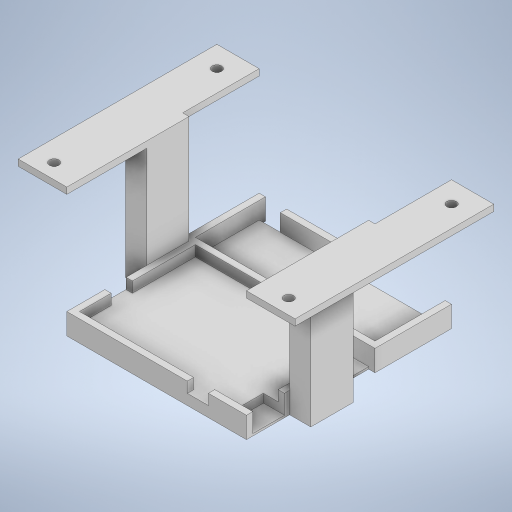
# Autodesk Inventor part: batter_pack_top
Saved by Autodesk Inventor 2023 (Build 270158000, 158)
## iProperties
Created: 2024-04-19
Part Number: batter_pack_top
Material: Genérico
Document SubType Name: Modeling
Designer: inigo
Density: 1 g/cm^3
Appearance: Valor por defecto
Author: inigo
Autodesk Inventor part; units mm, degrees
ref_plane "YZ Plane" through (0, 0, 0) normal (1, 0, 0) x (0, 1, 0)
ref_plane "XZ Plane" through (0, 0, 0) normal (0, 1, 0) x (-1, 0, 0)
ref_plane "XY Plane" through (0, 0, 0) normal (0, 0, 1) x (1, 0, 0)
sketch "Boceto1" plane through (0, 0, 0) normal (0, 1, 0) x (-1, 0, 0)
  line L0 (39.5, 42.5) -> (-39.5, 42.5)
  line L1 (-39.5, 42.5) -> (-39.5, -42.5)
  line L2 (-39.5, -42.5) -> (39.5, -42.5)
  line L3 (39.5, -42.5) -> (39.5, 42.5)
  line L4 (39.5, 42.5) -> (-39.5, -42.5) construction
  line L5 (-39.5, 42.5) -> (39.5, -42.5) construction
  line L6 (42.5, 45.5) -> (-42.5, 45.5)
  line L7 (-42.5, 45.5) -> (-42.5, -45.5)
  line L8 (-42.5, -45.5) -> (42.5, -45.5)
  line L9 (42.5, -45.5) -> (42.5, 45.5)
  point P0 (0, 0)
  point P1 (0, 0)
  dimension "d0" = 79
  dimension "d1" = 85
  dimension "d2" = 3
  constraints: 20 end point, 4 parallel, 2 midpoint, 2 perpendicular, 1 horizontal, 3 other
  measures "d0" distance of L2.end L1.end
  measures "d1" distance of L1.end L0.end
  measures "d2" distance between parallel lines of L3 L9
extrude "Extrusión1" add sketch "Boceto1" along normal blind 10 contours L3 L2 L1 L0 | L9 L8 L7 L6
sketch "Boceto2" plane through (0, 10, 0) normal (0, 1, 0) x (1, 0, 0)
  line L0 (-42.5, 45.5) -> (-42.5, -45.5)
  line L1 (42.5, -45.5) -> (-42.5, -45.5)
  line L2 (-42.5, -45.5) -> (-42.5, 45.5)
  line L3 (-42.5, 45.5) -> (42.5, 45.5)
  line L4 (42.5, 45.5) -> (42.5, -45.5)
  line L5 (42.5, -45.5) -> (-42.5, 45.5) construction
  line L6 (-42.5, -45.5) -> (42.5, 45.5) construction
  line L7 (-39.5, -42.5) -> (39.5, -42.5)
  line L8 (39.5, -42.5) -> (39.5, 42.5)
  line L9 (39.5, 42.5) -> (-39.5, 42.5)
  line L10 (-39.5, 42.5) -> (-39.5, -42.5)
  line L11 (0, -42.5) -> (0, -45.5)
  line L12 (-42.5, -45.5) -> (42.5, -45.5)
  line L13 (-15, -45.5) -> (15, -45.5)
  line L14 (15, -45.5) -> (15, -42.5)
  line L15 (15, -42.5) -> (-15, -42.5)
  line L16 (-15, -42.5) -> (-15, -45.5)
  line L17 (-15, -45.5) -> (15, -42.5) construction
  line L18 (15, -45.5) -> (-15, -42.5) construction
  line L19 (-65.3363, 15.3) -> (96.4695, 15.3)
  point P0 (0, 0)
  point P1 (0, -44)
  point P2 (39.5, 15.3)
  point P3 (-39.5, 15.3)
  dimension "d8" = 3
  dimension "d9" = 85
  dimension "d10" = 79
  dimension "d11" = 30
  dimension "d12" = 57.8
  constraints: 40 end point, 7 midpoint, 6 parallel, 3 horizontal, 3 perpendicular, 1 point on line, 3 other
  measures "d8" distance between parallel lines of L1 L7
  measures "d9" distance between parallel lines of L7 L9
  measures "d10" distance between parallel lines of L8 L10
  measures "d11" distance of L16.start L17.end
  measures "d12" distance between parallel lines of L7 L19
extrude "Extrusión2" cut sketch "Boceto2" against normal blind 5 contours L19 L8 L7 L10
sketch "Boceto3" plane through (0, 0, 0) normal (0, 1, 0) x (-1, 0, 0)
  line L0 (-42.5, 45.5) -> (-42.5, -15.3)
  line L1 (42.5, -45.5) -> (-42.5, -45.5)
  line L2 (-42.5, -45.5) -> (-42.5, -15.3)
  line L3 (-42.5, -15.3) -> (42.5, -15.3)
  line L4 (42.5, -15.3) -> (42.5, -45.5)
  line L5 (-45.5, -48.5) -> (45.5, -48.5)
  line L6 (45.5, -48.5) -> (45.5, -12.3)
  line L7 (45.5, -12.3) -> (-45.5, -12.3)
  line L8 (-45.5, -12.3) -> (-45.5, -48.5)
  line L9 (45.5, -15.3) -> (-45.5, -15.3)
  line L10 (-12.5, -48.5) -> (-12.5, -45.5)
  line L11 (-42.5, -45.5) -> (42.5, -45.5)
  line L12 (42.5, -45.5) -> (42.5, -48.5)
  line L13 (42.5, -15.3) -> (42.5, -12.3)
  line L14 (42.5, -45.5) -> (42.5, 45.5)
  line L15 (-42.5, -15.3) -> (-42.5, -12.3)
  line L16 (-42.5, 45.5) -> (-42.5, -45.5) projected
  line L17 (-42.5, -45.5) -> (-42.5, -48.5)
  line L18 (-42.5, -45.5) -> (42.5, -45.5) projected
  line L19 (2.5, -48.5) -> (32.5, -48.5)
  line L20 (32.5, -48.5) -> (32.5, -45.5)
  line L21 (32.5, -45.5) -> (2.5, -45.5)
  line L22 (2.5, -45.5) -> (2.5, -48.5)
  point P0 (0, 0)
  point P1 (0, 0)
  point P2 (-12.5, -47)
  point P3 (2.5, -45.5)
  point P4 (42.5, -47)
  point P5 (32.5, -47)
  dimension "d15" = 3
  dimension "d16" = 30
  dimension "d21" = 30
  dimension "d24" = 10
  constraints: 42 end point, 13 point on line, 6 parallel, 6 perpendicular, 3 midpoint, 2 horizontal, 3 other
  measures "d15" distance between parallel lines of L1 L5
  measures "d16" distance from line of L2 point (-12.5, -47)
  measures "d21" distance of L21.end L20.end
  measures "d24" distance of point (42.5, -47) point (32.5, -47)
extrude "Extrusión3" add sketch "Boceto3" along normal blind 10 contours L7 L13 L3 L0 | L0 L9 L8 L7 | L3 L4 L1 L2 | L2 L17 L5 L8 L9 | L7 L6 L9 L13 | L9 L6 L5 L12 L4 | L1 L20 L5 L22
sketch "Boceto4" plane through (0, 10, 0) normal (0, 1, 0) x (1, 0, 0)
  line L0 (-39.5, 15.3) -> (39.5, 15.3)
  line L1 (0, 15.3) -> (0, 45.5)
  line L2 (42.5, 45.5) -> (-42.5, 45.5)
  line L3 (-42.5, 45.5) -> (42.5, 45.5)
  line L4 (42.5, 45.5) -> (42.5, 15.3)
  line L5 (42.5, 15.3) -> (-42.5, 15.3)
  line L6 (-42.5, 15.3) -> (-42.5, 45.5)
  line L7 (-42.5, 45.5) -> (42.5, 15.3) construction
  line L8 (42.5, 45.5) -> (-42.5, 15.3) construction
  point P0 (0, 0)
  point P1 (0, 0)
  point P2 (0, 30.4)
  constraints: 18 end point, 5 midpoint, 2 parallel, 1 horizontal, 1 perpendicular
extrude "Extrusión4" cut sketch "Boceto4" against normal blind 8
sketch "Boceto5" plane through (-42.5, 0, 45.5) normal (-1, 0, 0) x (0, 0, 1)
  line L0 (-18, 10) -> (-28, 10)
  line L1 (-28, 10) -> (-28, 5)
  line L2 (-28, 5) -> (-18, 5)
  line L3 (-18, 5) -> (-18, 10)
  line L4 (-3, 5) -> (-57.8, 5) projected
  line L5 (-3, 10) -> (-3, 5) projected
  line L6 (-57.8, 10) -> (0, 10) projected
  point P0 (-45.5, 0)
  point P1 (-23, 5)
  dimension "d25" = 10
  dimension "d27" = 15
  dimension "d28" = 0
  dimension "d29" = 0
  constraints: 8 end point, 2 parallel, 1 horizontal, 1 perpendicular, 1 point on line
  measures "d25" distance of L2.end L1.end
  measures "d27" distance between parallel lines of L5 L3
  measures "d28" distance between parallel lines of L6 L0
  measures "d29" distance between parallel lines of L4 L2
extrude "Extrusión5" cut sketch "Boceto5" against normal blind 10 contours L3 L2 L1 L0
sketch "Boceto6" plane through (-42.5, 0, 45.5) normal (0, 0, 1) x (1, 0, 0)
  line L0 (67, 5) -> (57, 5)
  line L1 (57, 5) -> (57, 10)
  line L2 (57, 10) -> (67, 10)
  line L3 (67, 10) -> (67, 5)
  line L4 (82, 5) -> (3, 5) projected
  line L5 (85, 0) -> (85, 10) projected
  line L6 (0, 10) -> (85, 10) projected
  point P0 (42.5, 0)
  point P1 (62, 5)
  dimension "d32" = 10
  dimension "d33" = 18
  dimension "d34" = 0
  dimension "d35" = 0
  constraints: 8 end point, 2 parallel, 1 horizontal, 1 perpendicular, 1 point on line
  measures "d32" distance of L1.end L2.end
  measures "d33" distance between parallel lines of L5 L3
  measures "d34" distance between parallel lines of L6 L2
  measures "d35" distance between parallel lines of L4 L0
extrude "Extrusión6" cut sketch "Boceto6" against normal blind 10
sketch "Boceto7" plane through (42.5, 0, 45.5) normal (1, 0, 0) x (0, 0, -1)
  line L0 (57.8, 10) -> (3, 10) projected
  line L1 (3, 10) -> (18, 10)
  line L2 (18, 10) -> (18, 1)
  line L3 (18, 1) -> (3, 1)
  line L4 (3, 1) -> (3, 10)
  line L5 (3, 10) -> (3, 5) projected
  line L6 (57.8, 10) -> (28, 10) projected
  line L7 (57.8, 10) -> (42.8, 10)
  line L8 (42.8, 10) -> (42.8, 1)
  line L9 (42.8, 1) -> (57.8, 1)
  line L10 (57.8, 1) -> (57.8, 10)
  point P0 (45.5, 0)
  point P1 (0, 10)
  dimension "d41" = 15
  dimension "d42" = 9
  dimension "d43" = 0
  dimension "d46" = 15
  dimension "d47" = 9
  constraints: 16 end point, 4 parallel, 2 horizontal, 2 perpendicular, 1 point on line
  measures "d41" distance of L2.end L3.end
  measures "d42" distance of L1.end L2.end
  measures "d43" distance between parallel lines of L5 L4
  measures "d46" distance of L9.end L8.end
  measures "d47" distance of L8.end L7.end
extrude "Extrusión7" cut sketch "Boceto7" against normal blind 10
sketch "Boceto8" plane through (0, 0, 0) normal (0, 1, 0) x (-1, 0, 0)
  line L0 (42.5, -12.3) -> (42.5, 45.5) projected
  line L1 (42.5, -12.3) -> (52.5, -12.3)
  line L2 (52.5, -12.3) -> (52.5, 7.7)
  line L3 (52.5, 7.7) -> (42.5, 7.7)
  line L4 (42.5, 7.7) -> (42.5, -12.3)
  line L5 (45.5, -12.3) -> (42.5, -12.3) projected
  line L6 (-42.5, 45.5) -> (-42.5, -12.3) projected
  line L7 (-42.5, 5.1) -> (-52.5, 5.1)
  line L8 (-52.5, 5.1) -> (-52.5, 25.1)
  line L9 (-52.5, 25.1) -> (-42.5, 25.1)
  line L10 (-42.5, 25.1) -> (-42.5, 5.1)
  line L11 (-42.5, 2.7) -> (-39.5, 2.7) projected
  line L12 (-39.5, 27.5) -> (-42.5, 27.5) projected
  point P0 (0, 0)
  dimension "d48" = 10
  dimension "d49" = 20
  dimension "d50" = 0
  dimension "d51" = 10
  dimension "d52" = 20
  dimension "d53" = 2.4
  dimension "d54" = 2.4
  constraints: 16 end point, 4 parallel, 2 horizontal, 2 perpendicular, 2 point on line
  measures "d48" distance of L3.end L2.end
  measures "d49" distance of L2.end L1.end
  measures "d50" distance between parallel lines of L5 L1
  measures "d51" distance of L8.end L9.end
  measures "d52" distance of L7.end L8.end
  measures "d53" distance between parallel lines of L11 L7
  measures "d54" distance between parallel lines of L12 L9
extrude "Extrusión8" add sketch "Boceto8" along normal blind 58
sketch "Boceto9" plane through (0, 58, 0) normal (0, 1, 0) x (1, 0, 0)
  line L0 (-69.4566, 48.5) -> (100.0188, 48.5)
  line L1 (45.5, 48.5) -> (12.5, 48.5)
  line L2 (-42.5, -45.5) -> (42.5, -45.5)
  line L3 (-42.5, -45.5) -> (-83.2167, -45.5)
  line L4 (-83.2167, -45.5) -> (109.2502, -45.5)
  line L5 (65.5, 48.5) -> (65.5, -45.5)
  line L6 (45.5, 12.3) -> (45.5, 48.5)
  circle A0 centre (55.5, 38.5) radius 2.25
  line L7 (65.5, 0) -> (100.0188, 0)
  circle A1 centre (55.5, -38.5) radius 2.25
  line L8 (0, -45.5) -> (0, -59.2916)
  line L9 (-65.5, 48.5) -> (-65.5, -45.5)
  circle A2 centre (-55.5, -38.5) radius 2.25
  circle A3 centre (-55.5, 38.5) radius 2.25
  line L10 (-42.5, 12.3) -> (-42.5, -45.5)
  line L11 (-42.5, -45.5) -> (-42.5, 12.3)
  line L12 (-45.5, 12.3) -> (-42.5, 12.3)
  line L13 (-42.5, 12.3) -> (-45.5, 12.3)
  line L14 (-45.5, 48.5) -> (-45.5, 12.3)
  line L15 (-45.5, 12.3) -> (-45.5, 48.5)
  line L16 (-45.5, 48.5) -> (-65.5, 48.5)
  line L17 (42.5, 12.3) -> (45.5, 12.3)
  line L18 (45.5, 48.5) -> (45.5, 12.3)
  line L19 (45.5, 12.3) -> (42.5, 12.3)
  line L20 (15, -45.5) -> (42.5, -45.5)
  line L21 (42.5, 12.3) -> (42.5, -45.5)
  line L22 (42.5, -45.5) -> (65.5, -45.5)
  point P0 (0, 0)
  point P1 (0, 0)
  dimension "d57" = 20
  dimension "d58" = 4.5
  dimension "d59" = 10
  dimension "d60" = 10
  constraints: 46 end point, 5 perpendicular, 5 point on line, 5 symmetric about line, 4 centre point, 3 collinear, 3 other
  measures "d57" distance between parallel lines of L5 L6
  measures "d58" diameter of A0
  measures "d59" distance from line of L5 A0.centre
  measures "d60" distance from line of L0 A0.centre
extrude "Extrusión9" add sketch "Boceto9" along normal blind 3 contours L0 L14 L12 L10 L3 L9 | L0 L5 L4 L21 L17 L6
